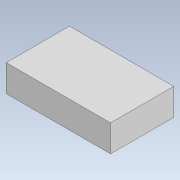
# Autodesk Inventor part: test
Saved by Autodesk Inventor 2020 (Build 240168000, 168)
## iProperties
Created: 2021-01-15
Part Number: test
Material: Generic
Document SubType Name: Modeling
Designer: DELL
Density: 1 g/cm^3
Appearance: Default
Author: DELL
Autodesk Inventor part; units mm, degrees
ref_plane "YZ Plane" through (0, 0, 0) normal (1, 0, 0) x (0, 1, 0)
ref_plane "XZ Plane" through (0, 0, 0) normal (0, 1, 0) x (-1, 0, 0)
ref_plane "XY Plane" through (0, 0, 0) normal (0, 0, 1) x (1, 0, 0)
sketch "Sketch1" plane through (0, 0, 0) normal (0, 1, 0) x (-1, 0, 0)
  line L0 (165, -100) -> (-165, -100)
  line L1 (-165, -100) -> (-165, 100)
  line L2 (-165, 100) -> (165, 100)
  line L3 (165, 100) -> (165, -100)
  line L4 (165, -100) -> (-165, 100) construction
  line L5 (-165, -100) -> (165, 100) construction
  point P0 (0, 0)
  dimension "d0" = 200
  dimension "d1" = 330
  constraints: 12 end point, 2 midpoint, 2 parallel, 1 horizontal, 1 perpendicular
  measures "d0" distance of L2.end L0.start
  measures "d1" distance of L1.end L2.end
extrude "Extrusion1" add sketch "Sketch1" along normal blind 85
body "Solid1"
